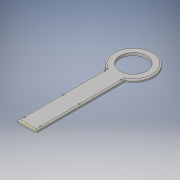
# Autodesk Inventor part: Arm Top Layer
Saved by Autodesk Inventor 2016 (Build 200138000, 138)
## iProperties
Created: 2016-04-22
Part Number: Arm Top Layer
Material: Generic
Document SubType Name: Modeling
Designer: rubenjm
Density: 1 g/cm^3
Appearance: Default
Author: rubenjm
Autodesk Inventor part; units mm, degrees
ref_plane "YZ Plane" through (0, 0, 0) normal (1, 0, 0) x (0, 1, 0)
ref_plane "XZ Plane" through (0, 0, 0) normal (0, 1, 0) x (-1, 0, 0)
ref_plane "XY Plane" through (0, 0, 0) normal (0, 0, 1) x (1, 0, 0)
sketch "Sketch1" plane through (0, 0, 0) normal (0, 1, 0) x (-1, 0, 0)
  arc A0 (44.4483, 506.0602) -> (-44.4517, 506.0602) centre (-0.0017, -1.4211) ccw construction
  arc A1 (44.4483, 506.0602) -> (-44.4517, 506.0602) centre (-0.0017, -1.4211) ccw
  line L0 (44.4483, 84.2454) -> (44.4483, 506.0602)
  line L1 (-44.4517, 506.0602) -> (-44.4517, 84.2454)
  circle A2 centre (-0.0017, 0.0032) radius 57.15 construction
  circle A3 centre (-0.0017, 0.0032) radius 63.5
  arc A4 (-44.4517, 84.2454) -> (44.4483, 84.2454) centre (-0.0017, 0.0032) ccw
  line L2 (-0.0017, 0.0032) -> (-0.0017, 508.0032) construction
  line L3 (-6.3517, -0.5116) -> (574.7506, -0.5116) construction
  point P0 (-7.0945, 251.5541)
  dimension "d19" = 88.9
  dimension "d29" = 114.3
  dimension "d30" = 127
  dimension "d31" = 190.5
  dimension "d32" = 508
  dimension "d35" = 88.9
  dimension "d38" = 90
  dimension "d40" = 90
  constraints: 8 end point, 7 point on circle, 5 centre point, 3 coincident, 1 concentric, 1 horizontal, 1 parallel
  measures "d19" distance of L1.start L0.end
  measures "d29" diameter of A2
  measures "d30" diameter of A3
  measures "d31" diameter of A4
  measures "d32" distance of L2.start L2.end
  measures "d35" distance between parallel lines of L1 L0
  measures "d38" angle of L2 L3
  measures "d40" angle of L3 L0
extrude "Extrusion2" add sketch "Sketch1" along normal blind 12.7
ref_plane "Work Plane3" through (44.4517, 12.7, 506.0602) normal (0, 0, -1) x (0, -1, 0)
sketch "Sketch2" plane through (0, 12.7, 0) normal (0, 1, 0) x (1, 0, 0)
  arc A0 (-44.4483, -506.0602) -> (44.4517, -506.0602) centre (0.0017, 1.4211) ccw construction
  line L0 (44.4517, -506.0602) -> (44.4517, -84.2454) construction
  line L1 (-44.4483, -506.0602) -> (44.4517, -506.0602) construction
  line L2 (44.4517, -506.0602) -> (44.4517, -84.2454) construction
  line L3 (44.4517, -84.2454) -> (-44.4483, -84.2454) construction
  line L4 (-44.4483, -84.2454) -> (-44.4483, -506.0602) construction
  line L5 (-44.4483, -84.2454) -> (-44.4483, -506.0602) construction
  line L6 (-44.4483, -295.1528) -> (-38.0983, -295.1528) construction
  line L7 (-38.0983, -295.1528) -> (-38.0983, -506.0602) construction
  line L8 (-38.0983, -295.1528) -> (-38.0983, -84.2454) construction
  circle A1 centre (-38.0983, -96.9454) radius 3.175
  circle A2 centre (-38.0983, -480.6602) radius 3.175
  circle A3 centre (-38.0983, -295.1528) radius 3.175
  line L9 (0.0017, -506.0602) -> (0.0017, 1.4211) construction
  line L10 (44.4517, -84.2454) -> (44.4517, -506.0602) construction
  line L11 (44.4517, -84.2454) -> (44.4517, -506.0602) construction
  line L12 (44.4517, -295.1528) -> (38.1017, -295.1528) construction
  line L13 (38.1017, -295.1528) -> (38.1017, -506.0602) construction
  line L14 (38.1017, -295.1528) -> (38.1017, -84.2454) construction
  circle A4 centre (38.1017, -96.9454) radius 3.175
  circle A5 centre (38.1017, -480.6602) radius 3.175
  circle A6 centre (38.1017, -295.1528) radius 3.175
  point P0 (0, 0)
  dimension "d41" = 6.35
  dimension "d42" = 90
  dimension "d43" = 6.35
  dimension "d44" = 12.7
  dimension "d45" = 6.35
  dimension "d46" = 6.35
  dimension "d49" = 25.4
  constraints: 26 end point, 8 symmetric about line, 6 centre point, 5 point on line, 2 coincident, 2 horizontal, 2 midpoint, 2 parallel, 1 perpendicular, 1 vertical, 3 other
  measures "d41" distance of L6.start L6.end
  measures "d42" angle of L6 L7
  measures "d43" diameter of A1
  measures "d44" distance from line of A1.centre L3
  measures "d45" diameter of A2
  measures "d46" diameter of A3
  measures "d49" distance of L7.end A2.centre
extrude "Extrusion3" cut sketch "Sketch2" against normal through all
sketch "Sketch3" plane through (0, 0, 0) normal (0, -1, 0) x (1, 0, 0)
  circle A0 centre (0.0017, 0.0032) radius 63.5 construction
  arc A1 (44.4517, 506.0602) -> (-44.4483, 506.0602) centre (0.0017, -1.4211) ccw construction
  line L0 (0.0017, 508.0032) -> (0.0017, 119.5102) construction
  line L1 (44.4517, 506.0602) -> (44.4517, 84.2454) construction
  line L2 (0.0017, 125.8602) -> (7.7487, 125.8602) construction
  line L3 (0.0017, 125.8602) -> (7.7487, 125.8602) construction
  line L4 (7.7487, 132.2102) -> (14.0987, 132.2102) construction
  line L5 (7.7487, 132.2102) -> (14.0987, 132.2102) construction
  line L6 (7.7487, 125.8602) -> (20.4487, 125.8602)
  line L7 (20.4487, 125.8602) -> (20.4487, 138.5602)
  line L8 (20.4487, 138.5602) -> (7.7487, 138.5602)
  line L9 (7.7487, 138.5602) -> (7.7487, 125.8602)
  line L10 (7.7487, 129.0352) -> (20.4487, 135.3852) construction
  line L11 (20.4487, 129.0352) -> (7.7487, 135.3852) construction
  line L12 (-7.7453, 132.2102) -> (-14.0953, 132.2102) construction
  line L13 (-7.7453, 132.2102) -> (-14.0953, 132.2102) construction
  line L14 (-7.7453, 125.8602) -> (-20.4453, 125.8602)
  line L15 (-20.4453, 125.8602) -> (-20.4453, 138.5602)
  line L16 (-20.4453, 138.5602) -> (-7.7453, 138.5602)
  line L17 (-7.7453, 138.5602) -> (-7.7453, 125.8602)
  point P0 (0, 0)
  point P1 (-20.4453, 135.3852)
  point P2 (-7.7453, 135.3852)
  dimension "d51" = 388.493
  dimension "d52" = 7.747
  dimension "d53" = 0
  dimension "d54" = 6.35
  dimension "d55" = 0
  dimension "d56" = 12.7
  dimension "d57" = 12.7
  dimension "d61" = 44.45
  constraints: 34 end point, 5 horizontal, 2 collinear, 2 midpoint, 2 parallel, 1 perpendicular, 1 point on circle, 1 vertical
  measures "d51" distance of L0.end L0.start
  measures "d52" distance of L2.start L2.end
  measures "d53" distance between parallel lines of L2 L3
  measures "d54" distance of L4.start L4.end
  measures "d55" distance between parallel lines of L4 L5
  measures "d56" distance of L8.end L7.end
  measures "d57" distance of L7.end L6.end
  measures "d61" distance from line of L1 L2.start
extrude "Extrusion4" cut sketch "Sketch3" against normal blind 6.35
fillet "Fillet1" radius 6.35 4 edges at (44.4517, 12.7, 295.1528) (-44.4483, 12.7, 295.1528) (0.0017, 12.7, 508.0032) (0.0017, 12.7, -95.2468)
equation "\"d35\" = d19"
body "Solid2"
